Autodesk Fusion 360 part; units mm, degrees
note: some values were not read from the file. Set by a fixed rule: which face or edge a step refers to.
(part 2 of 4)
sketch "Sketch34" plane through (0, 155, 0) normal (0, 1, 0) x (-1, 0, 0)
  line L0 (236, 20) -> (236, 10)
  line L1 (236, 10) -> (241, 10)
  line L2 (241, 10) -> (241, 15)
  line L3 (241, 15) -> (247, 15)
  line L4 (247, 15) -> (247, 10)
  line L5 (247, 10) -> (254, 10)
  line L6 (254, 10) -> (254, 51.2)
  line L7 (254, 51.2) -> (218, 51.2)
  line L8 (218, 51.2) -> (218, 42.3)
  line L9 (218, 42.3) -> (213, 42.3)
  line L10 (213, 42.3) -> (213, 37.3)
  line L11 (213, 37.3) -> (223, 37.3)
  line L12 (223, 37.3) -> (223, 20)
  line L13 (223, 20) -> (236, 20)
  line L14 (223, 20) -> (254, 20)
  line L15 (254, 20) -> (254, 51.2)
  line L16 (254, 51.2) -> (223, 51.2)
  line L17 (223, 51.2) -> (223, 20)
  line L18 (223, 51.2) -> (254, 51.2)
  line L19 (254, 51.2) -> (254, 46.2)
  line L20 (254, 46.2) -> (223, 46.2)
  line L21 (223, 46.2) -> (223, 51.2)
  line L22 (223, 20) -> (254, 20)
  line L23 (254, 20) -> (254, 30.7)
  line L24 (254, 30.7) -> (223, 30.7)
  line L25 (223, 30.7) -> (223, 20)
  line L26 (223, 51.2) -> (228.5, 51.2)
  line L27 (228.5, 51.2) -> (228.5, 20)
  line L28 (228.5, 20) -> (223, 20)
  line L29 (223, 20) -> (223, 51.2)
  line L30 (254, 51.2) -> (248.5, 51.2)
  line L31 (248.5, 51.2) -> (248.5, 20)
  line L32 (248.5, 20) -> (254, 20)
  line L33 (254, 20) -> (254, 51.2)
  dimension "d246" = 5
  dimension "d247" = 31
  dimension "d248" = 10.7
  dimension "d249" = 5.5
  dimension "d250" = 5.5
  constraint horizontal L14
  constraint vertical L15
  constraint horizontal L16
  constraint vertical L17
  constraint coincident L6.end L7.start
  constraint coincident L12.end L13.start
  constraint horizontal L18
  constraint vertical L19
  constraint horizontal L20
  constraint vertical L21
  constraint horizontal L22
  constraint vertical L23
  constraint horizontal L24
  constraint vertical L25
  constraint horizontal L26
  constraint vertical L27
  constraint horizontal L28
  constraint vertical L29
  constraint horizontal L30
  constraint vertical L31
  constraint horizontal L32
  constraint vertical L33
  measures "d246" distance of L16.end L20.end
  measures "d247" distance of L12.end L14.end
  measures "d248" distance of L12.end L24.end
  measures "d249" distance of L16.end L26.end
  measures "d250" distance of L6.end L30.end
extrude "Extrude92" cut sketch "Sketch34" against normal blind 2 contours L20 L24 L27 L31 bodies 1
sketch "Sketch35" plane through (0, 155, 0) normal (0, 1, 0) x (-1, 0, 0)
  line L0 (228.5, 46.2) -> (248.5, 46.2)
  line L1 (248.5, 46.2) -> (248.5, 30.7)
  line L2 (248.5, 30.7) -> (228.5, 30.7)
  line L3 (228.5, 30.7) -> (228.5, 46.2)
  line L4 (236, 20) -> (236, 10)
  line L5 (236, 10) -> (241, 10)
  line L6 (241, 10) -> (241, 15)
  line L7 (241, 15) -> (247, 15)
  line L8 (247, 15) -> (247, 10)
  line L9 (247, 10) -> (254, 10)
  line L10 (254, 10) -> (254, 51.2)
  line L11 (254, 51.2) -> (218, 51.2)
  line L12 (218, 51.2) -> (218, 42.3)
  line L13 (218, 42.3) -> (213, 42.3)
  line L14 (213, 42.3) -> (213, 37.3)
  line L15 (213, 37.3) -> (223, 37.3)
  line L16 (223, 37.3) -> (223, 20)
  line L17 (223, 20) -> (236, 20)
  line L18 (226.5, 48.2) -> (250.5, 48.2)
  line L19 (250.5, 48.2) -> (250.5, 28.7)
  line L20 (250.5, 28.7) -> (226.5, 28.7)
  line L21 (226.5, 28.7) -> (226.5, 48.2)
  dimension "d253" = -2
extrude "Extrude93" cut sketch "Sketch35" against normal blind 1 contours L18 L19 L20 L21 bodies 1
extrude "Extrude94" add 1 faces at (-236, 150, 36.1667) along direction (0, -1, 0) blind 5 on bodies 1 bodies 1
sketch "Sketch36" plane through (0, 153, 0) normal (0, 1, 0) x (-1, 0, 0)
  line L0 (248.5, 30.7) -> (248.5, 46.2)
  line L1 (248.5, 46.2) -> (228.5, 46.2)
  line L2 (228.5, 46.2) -> (228.5, 30.7)
  line L3 (228.5, 30.7) -> (248.5, 30.7)
  line L4 (228.5, 30.7) -> (248.5, 30.7)
  line L5 (248.5, 30.7) -> (248.5, 42.7)
  line L6 (248.5, 42.7) -> (228.5, 42.7)
  line L7 (228.5, 42.7) -> (228.5, 30.7)
  dimension "d258" = 12
  constraint horizontal L4
  constraint vertical L5
  constraint horizontal L6
  constraint vertical L7
  constraint coincident L2.end L3.start
  measures "d258" distance of L2.end L6.end
extrude "Extrude95" cut sketch "Sketch36" against normal blind 8 contours L0 L1 L2 L6 bodies 1
extrude "Extrude96" cut 1 faces at (-235.1667, 148, 46.2) along direction (0, 0, 1) blind 2 on bodies 1 bodies 1
extrude "Extrude97" cut 1 faces at (-235.1667, 148, 48.2) along direction (0, 0, 1) blind 3 on bodies 1 bodies 1
sketch "Sketch37" plane through (0, 153, 0) normal (0, 1, 0) x (-1, 0, 0)
  line L0 (248.5, 42.7) -> (228.5, 42.7)
  line L1 (228.5, 42.7) -> (228.5, 30.7)
  line L2 (228.5, 30.7) -> (248.5, 30.7)
  line L3 (248.5, 30.7) -> (248.5, 42.7)
  line L4 (228.5, 30.7) -> (230, 30.7)
  line L5 (230, 30.7) -> (230, 32.2)
  line L6 (230, 32.2) -> (228.5, 32.2)
  line L7 (228.5, 32.2) -> (228.5, 30.7)
  line L8 (248.5, 30.7) -> (247, 30.7)
  line L9 (247, 30.7) -> (247, 32.2)
  line L10 (247, 32.2) -> (248.5, 32.2)
  line L11 (248.5, 32.2) -> (248.5, 30.7)
  circle A0 centre (230, 32.2) radius 1.5
  circle A1 centre (247, 32.2) radius 1.5
  dimension "d265" = 1.5
  dimension "d266" = 1.5
  dimension "d267" = 1.5
  dimension "d268" = 1.5
  dimension "d269" = 3
  dimension "d270" = 3
  constraint horizontal L4
  constraint vertical L5
  constraint horizontal L6
  constraint vertical L7
  constraint coincident L1.end L2.start
  constraint horizontal L8
  constraint vertical L9
  constraint horizontal L10
  constraint vertical L11
  constraint coincident L2.end L3.start
  constraint coincident L5.end L6.start
  constraint coincident L9.end L10.start
  measures "d265" distance of L1.end L4.end
  measures "d266" distance of L1.end L6.end
  measures "d267" distance of L2.end L8.end
  measures "d268" distance of L2.end L10.end
  measures "d269" diameter of A0
  measures "d270" diameter of A1
extrude "Extrude98" cut sketch "Sketch37" against normal blind 8 contours L9 L10 A1 | L9 L10 A1 | L5 L6 A0 | L5 L6 A0 bodies 1
extrude "Extrude99" cut 1 faces at (-241.8333, 154, 29.3667) along direction (0, -1, 0) blind 4 on bodies 1 bodies 1
extrude "Extrude100" cut 1 faces at (-236.0332, 153, 39.5401) along direction (0, -1, 0) blind 3 on bodies 1 bodies 1
extrude "Extrude101" cut 1 faces at (-248.2053, 153, 30.9947) along direction (0, -1, 0) blind 3 on bodies 1 bodies 1
extrude "Extrude102" cut 1 faces at (-228.7947, 153, 30.9947) along direction (0, -1, 0) blind 3 on bodies 1 bodies 1
sketch "Sketch38" plane through (0, 150, 0) normal (0, 1, 0) x (-1, 0, 0)
  circle A0 centre (247, 32.2) radius 1.5
  circle A1 centre (230, 32.2) radius 1.5
  line L0 (248.5, 42.7) -> (228.5, 42.7)
  line L1 (228.5, 42.7) -> (228.5, 51.2)
  line L2 (228.5, 51.2) -> (226.5, 51.2)
  line L3 (226.5, 51.2) -> (226.5, 28.7)
  line L4 (226.5, 28.7) -> (250.5, 28.7)
  line L5 (250.5, 28.7) -> (250.5, 51.2)
  line L6 (250.5, 51.2) -> (248.5, 51.2)
  line L7 (248.5, 51.2) -> (248.5, 42.7)
  circle A2 centre (230, 32.2) radius 2.5
  circle A3 centre (247, 32.2) radius 2.5
  dimension "d281" = 1
  dimension "d282" = 1
extrude "Extrude103" add sketch "Sketch38" along normal blind 1 contours A2 | A3 bodies 1
extrude "Extrude104" add 1 faces at (-237.6667, 145, 27.6994) along direction (0, -1, 0) blind 10 on bodies 1 bodies 1
extrude "Extrude105" cut 1 faces at (-240.8138, 150, 39.8515) along direction (0, -1, 0) blind 5 on bodies 1 bodies 1
extrude "Extrude106" cut 1 faces at (-240.8138, 145, 39.8515) along direction (0, -1, 0) blind 3 on bodies 1 bodies 1
extrude "Extrude107" cut 1 faces at (-229.0289, 151, 34.1304) along direction (0, -1, 0) blind 5 on bodies 1 bodies 1
extrude "Extrude108" cut 1 faces at (-246.0289, 151, 30.2696) along direction (0, -1, 0) blind 5 on bodies 1 bodies 1
extrude "Extrude109" add 1 faces at (-70.3333, 62, -59.3333) along direction (0, -1, 0) blind 27 on bodies 1 bodies 1
extrude "Extrude110" add 1 faces at (-240.3333, 62, -59.3333) along direction (0, -1, 0) blind 27 on bodies 1 bodies 1
sketch "Sketch39" plane through (0, 0, -61) normal (0, 0, 1) x (1, 0, 0)
  line L0 (-249, 5) -> (-66, 5)
  line L1 (-66, 5) -> (-66, 35)
  line L2 (-66, 35) -> (-79, 35)
  line L3 (-79, 35) -> (-236, 35)
  line L4 (-236, 35) -> (-249, 35)
  line L5 (-249, 35) -> (-249, 5)
  line L6 (-249, 5) -> (-236, 5)
  line L7 (-236, 5) -> (-236, 35)
  line L8 (-236, 35) -> (-249, 35)
  line L9 (-249, 35) -> (-249, 5)
  constraint horizontal L6
  constraint vertical L7
  constraint horizontal L8
  constraint vertical L9
  constraint coincident L3.end L4.start
  constraint coincident L0.start L5.end
extrude "Extrude111" add sketch "Sketch39" along normal blind 5 contours L0 L4 L5 L6 L7 L8 L9 bodies 1
sketch "Sketch40" plane through (0, 0, -61) normal (0, 0, 1) x (1, 0, 0)
  line L0 (-236, 35) -> (-236, 5)
  line L1 (-236, 5) -> (-66, 5)
  line L2 (-66, 5) -> (-66, 35)
  line L3 (-66, 35) -> (-79, 35)
  line L4 (-79, 35) -> (-236, 35)
  line L5 (-66, 5) -> (-79, 5)
  line L6 (-79, 5) -> (-79, 35)
  line L7 (-79, 35) -> (-66, 35)
  line L8 (-66, 35) -> (-66, 5)
  constraint horizontal L5
  constraint vertical L6
  constraint horizontal L7
  constraint vertical L8
  constraint coincident L3.end L4.start
  constraint coincident L1.end L2.start
extrude "Extrude112" add sketch "Sketch40" along normal blind 5 contours L1 L2 L3 L5 L6 L7 L8 bodies 1
extrude "Extrude113" add 1 faces at (-74.6667, 62, 13.3333) along direction (0, -1, 0) blind 57 on bodies 1 bodies 1
sketch "Sketch41" plane through (0, 60.5, 0) normal (0, -1, 0) x (1, 0, 0)
  line L0 (-223, 37.3) -> (-213, 37.3)
  line L1 (-213, 37.3) -> (-213, 45.2)
  line L2 (-213, 45.2) -> (-102, 45.2)
  line L3 (-102, 45.2) -> (-102, 37.3)
  line L4 (-102, 37.3) -> (-92, 37.3)
  line L5 (-92, 37.3) -> (-92, 51.2)
  line L6 (-92, 51.2) -> (-223, 51.2)
  line L7 (-223, 51.2) -> (-223, 37.3)
  line L8 (-92, 51.2) -> (-102, 51.2)
  line L9 (-102, 51.2) -> (-102, 37.3)
  line L10 (-102, 37.3) -> (-92, 37.3)
  line L11 (-92, 37.3) -> (-92, 51.2)
  constraint horizontal L8
  constraint vertical L9
  constraint horizontal L10
  constraint vertical L11
  constraint coincident L3.end L4.start
  constraint coincident L5.end L6.start
extrude "Extrude114" add sketch "Sketch41" along normal blind 2 contours L3 L4 L5 L6 L8 L9 L10 L11 bodies 1
extrude "Extrude115" add 1 faces at (-98.6667, 58.5, 41.9333) along direction (0, -1, 0) blind 53.5 on bodies 1 bodies 1
sketch "Sketch42" plane through (0, 60.5, 0) normal (0, -1, 0) x (1, 0, 0)
  line L0 (-102, 45.2) -> (-102, 51.2)
  line L1 (-102, 51.2) -> (-223, 51.2)
  line L2 (-223, 51.2) -> (-223, 37.3)
  line L3 (-223, 37.3) -> (-213, 37.3)
  line L4 (-213, 37.3) -> (-213, 45.2)
  line L5 (-213, 45.2) -> (-102, 45.2)
  line L6 (-223, 51.2) -> (-213, 51.2)
  line L7 (-213, 51.2) -> (-213, 37.3)
  line L8 (-213, 37.3) -> (-223, 37.3)
  line L9 (-223, 37.3) -> (-223, 51.2)
  line L10 (-213, 51.2) -> (-218, 51.2)
  line L11 (-218, 51.2) -> (-218, 37.3)
  line L12 (-218, 37.3) -> (-213, 37.3)
  line L13 (-213, 37.3) -> (-213, 51.2)
  constraint horizontal L6
  constraint vertical L7
  constraint horizontal L8
  constraint vertical L9
  constraint coincident L3.end L4.start
  constraint coincident L1.end L2.start
  constraint horizontal L10
  constraint vertical L11
  constraint horizontal L12
  constraint vertical L13
  constraint midpoint L3 L11.end
extrude "Extrude116" add sketch "Sketch42" along normal blind 55.5 contours L1 L3 L4 L6 L7 L8 L10 L11 L12 L13 bodies 1
extrude "Extrude117" add 1 faces at (-240.3333, 62, 13.3333) along direction (0, -1, 0) blind 57 on bodies 1 bodies 1
extrude "Extrude118" cut 1 faces at (-228.5, 139.6667, 48.3667) along direction (1, 0, 0) blind 2 on bodies 1 bodies 1
extrude "Extrude119" cut 1 faces at (-248.5, 137.3333, 48.3667) along direction (-1, 0, 0) blind 2 on bodies 1 bodies 1
extrude "Extrude120" cut 1 faces at (-249, 48.3333, 37.9667) along direction (-1, 0, 0) blind 1.5 on bodies 1 bodies 1
sketch "Sketch43" plane through (0, 0, -66) normal (0, 0, -1) x (-1, 0, 0)
  line L0 (56, 160) -> (56, 0)
  line L1 (56, 0) -> (259, 0)
  line L2 (259, 0) -> (259, 160)
  line L3 (259, 160) -> (254, 160)
  line L4 (254, 160) -> (254, 155)
  line L5 (254, 155) -> (236, 155)
  line L6 (236, 155) -> (236, 35)
  line L7 (236, 35) -> (79, 35)
  line L8 (79, 35) -> (79, 155)
  line L9 (79, 155) -> (61, 155)
  line L10 (61, 155) -> (61, 160)
  line L11 (61, 160) -> (56, 160)
extrude "Extrude121" add sketch "Sketch43" along normal blind 5 bodies 1
sketch "Sketch44" plane through (0, 35, 0) normal (0, 1, 0) x (-1, 0, 0)
  line L0 (236, -71) -> (236, -61)
  line L1 (236, -61) -> (79, -61)
  line L2 (79, -61) -> (79, -71)
  line L3 (79, -71) -> (236, -71)
  line L4 (79, -61) -> (236, -61)
  line L5 (236, -61) -> (236, -66)
  line L6 (236, -66) -> (79, -66)
  line L7 (79, -66) -> (79, -61)
  constraint horizontal L4
  constraint vertical L5
  constraint horizontal L6
  constraint vertical L7
  constraint midpoint L0 L5.end
  constraint coincident L1.end L2.start
extrude "Extrude122" cut sketch "Sketch44" against normal blind 10 contours L0 L2 L3 L6 bodies 1
sketch "Sketch45" plane through (0, 0, 0) normal (0, -1, 0) x (1, 0, 0)
  circle A0 through (-148, -53.875, -5) (-154, -50.4109, -5) (-154, -57.3391, -5)
  circle A1 through (-159, -12.125, -5) (-165, -8.6609, -5) (-165, -15.5891, -5)
sketch "Sketch46" plane through (0, 0, 56.2) normal (0, 0, 1) x (1, 0, 0)
  circle A0 centre (-229, 25) radius 5.65
  circle A1 centre (-157.5, 25) radius 5.5
  line L0 (-259, 5) -> (-272.5, 5)
  line L1 (-272.5, 5) -> (-272.5, 0)
  line L2 (-272.5, 0) -> (-42.5, 0)
  line L3 (-42.5, 0) -> (-42.5, 5)
  line L4 (-42.5, 5) -> (-56, 5)
  line L5 (-56, 5) -> (-56, 160)
  line L6 (-56, 160) -> (-259, 160)
  line L7 (-259, 160) -> (-259, 5)
  circle A2 centre (-229, 25) radius 6.15
  circle A3 centre (-157.5, 25) radius 6.15
  dimension "d323" = 12.3
  dimension "d324" = 12.3
  constraint concentric A0 A2
  constraint concentric A1 A3
  measures "d323" diameter of A2
  measures "d324" diameter of A3
extrude "Extrude123" cut sketch "Sketch46" against normal blind 5 contours A2 | A3 bodies 1
extrude "Extrude124" cut 1 faces at (-183.6667, 15, -61) along direction (0, 0, -1) blind 3 on bodies 1 bodies 1
extrude "Extrude125" cut 1 faces at (-102, 23.5, 44.5667) along direction (1, 0, 0) blind 0.5 on bodies 1 bodies 1
extrude "Extrude126" cut 1 faces at (-213, 23.5, 44.5667) along direction (-1, 0, 0) blind 0.5 on bodies 1 bodies 1
extrude "Extrude127" cut 1 faces at (-215, 95.3333, 42.3) along direction (0, 0, -1) blind 0.5 on bodies 1 bodies 1
extrude "Extrude128" cut 1 faces at (-100, 125.1667, 42.3) along direction (0, 0, -1) blind 0.5 on bodies 1 bodies 1
sketch "Sketch47" plane through (0, 0, -71) normal (0, 0, -1) x (-1, 0, 0)
  line L0 (236, 155) -> (236, 25)
  line L1 (236, 25) -> (79, 25)
  line L2 (79, 25) -> (79, 155)
  line L3 (79, 155) -> (61, 155)
  line L4 (61, 155) -> (61, 160)
  line L5 (61, 160) -> (56, 160)
  line L6 (56, 160) -> (56, 0)
  line L7 (56, 0) -> (259, 0)
  line L8 (259, 0) -> (259, 160)
  line L9 (259, 160) -> (254, 160)
  line L10 (254, 160) -> (254, 155)
  line L11 (254, 155) -> (236, 155)
  line L12 (61, 155) -> (79, 155)
  line L13 (79, 155) -> (79, 25)
  line L14 (79, 25) -> (61, 25)
  line L15 (61, 25) -> (61, 155)
  line L16 (236, 25) -> (254, 25)
  line L17 (254, 25) -> (254, 155)
  line L18 (254, 155) -> (236, 155)
  line L19 (236, 155) -> (236, 25)
  constraint horizontal L12
  constraint vertical L13
  constraint horizontal L14
  constraint vertical L15
  constraint coincident L1.end L2.start
  constraint coincident L3.end L4.start
  constraint horizontal L16
  constraint vertical L17
  constraint horizontal L18
  constraint vertical L19
  constraint coincident L10.end L11.start
  constraint coincident L0.end L1.start
extrude "Extrude129" cut sketch "Sketch47" against normal blind 5 contours L0 L11 L16 L17 L18 L19 | L2 L3 L12 L13 L14 L15 bodies 1
extrude "Extrude130" cut 1 faces at (-97, 95.3333, 44.9333) along direction (1, 0, 0) blind 1 on bodies 1 bodies 1
extrude "Extrude131" cut 1 faces at (-218, 95.3333, 44.9333) along direction (-1, 0, 0) blind 1 on bodies 1 bodies 1
extrude "Extrude132" add 1 faces at (-92, 105, 41.9333) along direction (1, 0, 0) blind 3 on bodies 1 bodies 1
extrude "Extrude133" cut 1 faces at (-138.8333, 65.5, 49.2) along direction (0, -1, 0) blind 1 on bodies 1 bodies 1
extrude "Extrude134" add 1 faces at (-138.8333, 60.5, 49.2) along direction (0, -1, 0) blind 1 on bodies 1 bodies 1
extrude "Extrude135" cut 1 faces at (-70, 125.6667, 15) along direction (0, 0, 1) blind 0.5 on bodies 1 bodies 1
extrude "Extrude136" cut 1 faces at (-70, 96.3333, -61) along direction (0, 0, -1) blind 0.5 on bodies 1 bodies 1
extrude "Extrude137" cut 1 faces at (-245, 96.3333, 15) along direction (0, 0, 1) blind 0.5 on bodies 1 bodies 1
extrude "Extrude138" cut 1 faces at (-243, 128.3333, -61) along direction (0, 0, -1) blind 0.5 on bodies 1 bodies 1
sketch "Sketch48" plane through (0, 5, 0) normal (0, 1, 0) x (-1, 0, 0)
  line L0 (101.5, 37.3) -> (89, 37.3)
  line L1 (89, 37.3) -> (89, 51.2)
  line L2 (89, 51.2) -> (66, 51.2)
  line L3 (66, 51.2) -> (66, 20)
  line L4 (66, 20) -> (79, 20)
  line L5 (79, 20) -> (79, 10)
  line L6 (79, 10) -> (66, 10)
  line L7 (66, 10) -> (66, -20)
  line L8 (66, -20) -> (249, -20)
  line L9 (249, -20) -> (249, 10)
  line L10 (249, 10) -> (236, 10)
  line L11 (236, 10) -> (236, 20)
  line L12 (236, 20) -> (250.5, 20)
  line L13 (250.5, 20) -> (250.5, 51.2)
  line L14 (250.5, 51.2) -> (218, 51.2)
  line L15 (218, 51.2) -> (218, 37.3)
  line L16 (218, 37.3) -> (213.5, 37.3)
  line L17 (213.5, 37.3) -> (213.5, 51.2)
  line L18 (213.5, 51.2) -> (185, 51.2)
  line L19 (185, 51.2) -> (185, 3)
  line L20 (185, 3) -> (130, 3)
  line L21 (130, 3) -> (130, 51.2)
  line L22 (130, 51.2) -> (101.5, 51.2)
  line L23 (101.5, 51.2) -> (101.5, 37.3)
  circle A0 centre (163, -12.125) radius 4
extrude "Extrude139" add 1 faces at (-42.5, 3.3333, 38.4667) along direction (1, 0, 0) blind 42.5 on bodies 1 bodies 1
extrude "Extrude140" add 1 faces at (-272.5, 1.6667, 20.7333) along direction (-1, 0, 0) blind 42.5 on bodies 1 bodies 1
sketch "Sketch49" plane through (0, 0, 3) normal (0, 0, -1) x (-1, 0, 0)
  line L0 (259, 0) -> (185, 0)
  line L1 (185, 0) -> (185, -3)
  line L2 (185, -3) -> (270, -3)
  line L3 (270, -3) -> (270, 0)
  line L4 (270, 0) -> (315, 0)
  line L5 (315, 0) -> (315, 5)
  line L6 (315, 5) -> (259, 5)
  line L7 (259, 5) -> (259, 0)
  line L8 (259, 5) -> (315, 5)
  line L9 (315, 5) -> (315, 0)
  line L10 (315, 0) -> (259, 0)
  line L11 (259, 0) -> (259, 5)
  constraint horizontal L8
  constraint vertical L9
  constraint horizontal L10
  constraint vertical L11
  constraint coincident L4.end L5.start
  constraint coincident L6.end L7.start
extrude "Extrude141" add sketch "Sketch49" along normal blind 3 contours L4 L5 L6 L7 L8 L9 L10 L11 bodies 1
sketch "Sketch50" plane through (0, 0, 3) normal (0, 0, -1) x (-1, 0, 0)
  line L0 (45, 0) -> (45, -3)
  line L1 (45, -3) -> (130, -3)
  line L2 (130, -3) -> (130, 0)
  line L3 (130, 0) -> (56, 0)
  line L4 (56, 0) -> (56, 5)
  line L5 (56, 5) -> (0, 5)
  line L6 (0, 5) -> (0, 0)
  line L7 (0, 0) -> (45, 0)
  line L8 (56, 5) -> (0, 5)
  line L9 (0, 5) -> (0, 0)
  line L10 (0, 0) -> (56, 0)
  line L11 (56, 0) -> (56, 5)
  constraint horizontal L8
  constraint vertical L9
  constraint horizontal L10
  constraint vertical L11
  constraint coincident L6.end L7.start
  constraint coincident L4.end L5.start
extrude "Extrude142" add sketch "Sketch50" along normal blind 3 contours L4 L5 L6 L7 L8 L9 L10 L11 bodies 1
sketch "Sketch51" plane through (0, 5, 0) normal (0, 1, 0) x (-1, 0, 0)
  line L0 (56, 0) -> (56, 56.2)
  line L1 (56, 56.2) -> (0, 56.2)
  line L2 (0, 56.2) -> (0, 0)
  line L3 (0, 0) -> (56, 0)
  line L4 (56, 56.2) -> (0, 0)
  line L5 (56, 56.2) -> (0, 56.2)
  line L6 (0, 56.2) -> (0, 0)
  constraint coincident L0.end L1.start
  constraint coincident L2.end L3.start
  constraint coincident L1.end L2.start
extrude "Extrude143" cut sketch "Sketch51" against normal blind 5 contours L1 L2 L4 L5 L6 bodies 1
sketch "Sketch52" plane through (0, 5, 0) normal (0, 1, 0) x (-1, 0, 0)
  line L0 (315, 0) -> (315, 56.2)
  line L1 (315, 56.2) -> (259, 56.2)
  line L2 (259, 56.2) -> (259, 0)
  line L3 (259, 0) -> (315, 0)
  line L4 (315, 0) -> (259, 56.2)
  line L5 (315, 0) -> (315, 56.2)
  line L6 (315, 56.2) -> (259, 56.2)
  constraint coincident L0.start L3.end
  constraint coincident L1.end L2.start
  constraint coincident L0.end L1.start
extrude "Extrude144" cut sketch "Sketch52" against normal blind 5 contours L0 L1 L4 L5 L6 bodies 1
sketch "Sketch53" plane through (0, 0, 0) normal (0, -1, 0) x (1, 0, 0)
sketch "Sketch54" plane through (0, 5, 0) normal (0, 1, 0) x (-1, 0, 0)
  line L0 (56, 56.2) -> (0, 0)
  line L1 (0, 0) -> (56, 0)
  line L2 (56, 0) -> (56, 56.2)
  line L3 (45, 45.1607, -5) -> (45, 51.2, -5)
  line L4 (45, 51.2, -5) -> (45, 51.2, 0)
  line L5 (45, 51.2) -> (45, 45.1607)
  line L6 (45, 45.1607, 0) -> (45, 45.1607, -5)
  point P0 (45, 45.1607)
  dimension "d369" = 5
  constraint vertical L5
  constraint coincident P0 L5.end
  measures "d369" distance of P0 L5.end
extrude "Extrude145" cut sketch "Sketch54" along normal blind 6 contours L3 L4 L5 L6 in plane through (-45, 5, 0) normal (-1, 0, 0) bodies 1
extrude "Extrude146" add 1 faces at (-47, 3.3333, 45.1607) along direction (0, 0, 1) blind 11 on bodies 1 bodies 1
sketch "Sketch55" plane through (0, 5, 0) normal (0, 1, 0) x (-1, 0, 0)
  line L0 (51, 51.1821) -> (51, 56.1607)
  line L1 (51, 56.1607) -> (45, 56.1607)
  line L2 (45, 56.1607) -> (45, 45.1607)
  line L3 (45, 45.1607) -> (0, 0)
  line L4 (0, 0) -> (56, 0)
  line L5 (56, 0) -> (56, 56.2)
  line L6 (56, 56.2) -> (51, 51.1821)
  line L7 (56, 56.2) -> (51, 56.1607)
  line L8 (51, 51.1821) -> (56, 56.2)
  line L9 (51, 56.1607) -> (51, 51.1821)
  constraint coincident L5.end L6.start
  constraint coincident L0.end L1.start
  constraint coincident L0.start L6.end
extrude "Extrude147" add sketch "Sketch55" against normal blind 5 contours L0 L6 L7 L8 L9 bodies 1
sketch "Sketch56" plane through (-158.0615, 0, 157.499) normal (-0.708366, 0, 0.705845) x (0.705845, 0, 0.708366)
  line L0 (-143.0037, 5) -> (-222.3412, 5)
  line L1 (-222.3412, 5) -> (-222.3412, 0)
  line L2 (-222.3412, 0) -> (-158.5879, 0)
  line L3 (-158.5879, 0) -> (-150.0622, 0)
  line L4 (-150.0622, 0) -> (-143.0037, 0)
  line L5 (-143.0037, 0) -> (-143.0037, 5)
  line L6 (-158.5879, 0, 0) -> (-154.3099, 0, 4.2628)
  line L7 (-154.3099, 0, 4.2628) -> (-150.0622, 0, 0)
  line L8 (-158.5879, 0) -> (-150.0622, 0)
  line L9 (-150.0622, 0) -> (-158.5879, 0)
  line L10 (-158.5879, 0) -> (-158.5879, 5)
  line L11 (-158.5879, 5) -> (-150.0622, 5)
  line L12 (-150.0622, 5) -> (-150.0622, 0)
  point P0 (-154.3099, 0)
  constraint coincident L2.end L3.start
  constraint coincident L3.end L4.start
  constraint horizontal L9
  constraint vertical L10
  constraint horizontal L11
  constraint vertical L12
  constraint coincident L0 L10.end
extrude "Extrude148" add sketch "Sketch56" along normal blind 5 contours L3 L6 L7 L8 L9 in plane through (-158.0615, 0, 157.499) normal (0, 1, 0) bodies 1
sketch "Sketch57" plane through (0, 5, 0) normal (0, 1, 0) x (-1, 0, 0)
  line L0 (315, 0) -> (270, 45.1607)
  line L1 (270, 45.1607) -> (270, 51.2)
  line L2 (270, 51.2) -> (263.9822, 51.2)
  line L3 (263.9822, 51.2) -> (259, 56.2)
  line L4 (259, 56.2) -> (259, 0)
  line L5 (259, 0) -> (315, 0)
  line L6 (259, 56.2) -> (270, 56.2)
  line L7 (270, 56.2) -> (270, 51.2)
  line L8 (270, 51.2) -> (259, 51.2)
  line L9 (259, 51.2) -> (259, 56.2)
  line L10 (259, 56.2) -> (263.9822, 51.2)
  constraint horizontal L6
  constraint vertical L7
  constraint horizontal L8
  constraint vertical L9
  constraint coincident L1.end L2.start
  constraint coincident L3.end L4.start
  constraint coincident L2.end L3.start
extrude "Extrude149" add sketch "Sketch57" against normal blind 5 contours L2 L3 L6 L7 L8 L10 bodies 1
extrude "Extrude150" add 1 faces at (-33.6667, 5, 15.0536) along direction (0, 1, 0) blind 155 on bodies 1 bodies 1
extrude "Extrude151" add 1 faces at (-281.3333, 5, 15.0536) along direction (0, 1, 0) blind 155 on bodies 1 bodies 1
extrude "Extrude152" cut 1 faces at (-243, 67, 11.8333) along direction (0, -1, 0) blind 5 on bodies 1 bodies 1
extrude "Extrude153" cut 1 faces at (-245, 75, -59.6667) along direction (0, -1, 0) blind 5 on bodies 1 bodies 1
extrude "Extrude154" cut 1 faces at (-72, 67, 11.8333) along direction (0, -1, 0) blind 5 on bodies 1 bodies 1
extrude "Extrude155" cut 1 faces at (-72, 67, -59.6667) along direction (0, -1, 0) blind 5 on bodies 1 bodies 1
extrude "Extrude156" add 1 faces at (-63.3333, 155, -61.1667) along direction (0, 1, 0) blind 62 on bodies 1 bodies 1
extrude "Extrude157" add 1 faces at (-251.6667, 155, -61.1667) along direction (0, 1, 0) blind 62 on bodies 1 bodies 1
sketch "Sketch58" plane through (0, 155, 0) normal (0, 1, 0) x (-1, 0, 0)
  line L0 (68, 10) -> (68, 15.5)
  line L1 (68, 15.5) -> (74, 15.5)
  line L2 (74, 15.5) -> (74, 10)
  line L3 (74, 10) -> (79, 10)
  line L4 (79, 10) -> (79, 20)
  line L5 (79, 20) -> (66, 20)
  line L6 (66, 20) -> (66, 51.2)
  line L7 (66, 51.2) -> (61, 51.2)
  line L8 (61, 51.2) -> (61, 10)
  line L9 (61, 10) -> (68, 10)
  line L10 (79, 20) -> (61, 20)
  line L11 (61, 20) -> (61, 15.5)
  line L12 (61, 15.5) -> (79, 15.5)
  line L13 (79, 15.5) -> (79, 20)
  constraint horizontal L10
  constraint vertical L11
  constraint horizontal L12
  constraint vertical L13
  constraint coincident L8 L11.end
  constraint coincident L4.end L5.start
extrude "Extrude158" add sketch "Sketch58" along normal blind 62 contours L0 L8 L9 L12 | L1 L4 L5 L8 L10 L11 L12 L13 | L2 L3 L4 L12 bodies 1
sketch "Sketch59" plane through (0, 155, 0) normal (0, 1, 0) x (-1, 0, 0)
  line L0 (241, 10) -> (241, 15.5)
  line L1 (241, 15.5) -> (247, 15.5)
  line L2 (247, 15.5) -> (247, 10)
  line L3 (247, 10) -> (254, 10)
  line L4 (254, 10) -> (254, 51.2)
  line L5 (254, 51.2) -> (250.5, 51.2)
  line L6 (250.5, 51.2) -> (250.5, 28.7)
  line L7 (250.5, 28.7) -> (226.5, 28.7)
  line L8 (226.5, 28.7) -> (226.5, 51.2)
  line L9 (226.5, 51.2) -> (219, 51.2)
  line L10 (219, 51.2) -> (219, 41.8)
  line L11 (219, 41.8) -> (213.5, 41.8)
  line L12 (213.5, 41.8) -> (213.5, 37.3)
  line L13 (213.5, 37.3) -> (223, 37.3)
  line L14 (223, 37.3) -> (223, 20)
  line L15 (223, 20) -> (236, 20)
  line L16 (236, 20) -> (236, 10)
  line L17 (236, 10) -> (241, 10)
  line L18 (236, 20) -> (254, 20)
  line L19 (254, 20) -> (254, 15.5)
  line L20 (254, 15.5) -> (236, 15.5)
  line L21 (236, 15.5) -> (236, 20)
  constraint horizontal L18
  constraint vertical L19
  constraint horizontal L20
  constraint vertical L21
  constraint coincident L4 L19.end
  constraint coincident L15.end L16.start
extrude "Extrude159" add sketch "Sketch59" along normal blind 62 contours L0 L16 L17 L20 | L1 L4 L16 L18 L19 L20 L21 | L2 L3 L4 L20 bodies 1
extrude "Extrude160" add 1 faces at (-33.6667, 160, 15.0536) along direction (0, 1, 0) blind 65 on bodies 1 bodies 1
sketch "Sketch60" plane through (0, 225, 0) normal (0, 1, 0) x (-1, 0, 0)
  line L0 (270, 56.2) -> (56, 56.2)
  line L1 (56, 56.2) -> (51, 56.1607)
  line L2 (51, 56.1607) -> (45, 56.1607)
  line L3 (45, 56.1607) -> (45, 45.1607)
  line L4 (45, 45.1607) -> (0, 0)
  line L5 (0, 0) -> (56, 0)
  line L6 (56, 0) -> (56, -71)
  line L7 (56, -71) -> (61, -71)
  line L8 (61, -71) -> (61, 51.2)
  line L9 (61, 51.2) -> (254, 51.2)
  line L10 (254, 51.2) -> (254, -71)
  line L11 (254, -71) -> (259, -71)
  line L12 (259, -71) -> (259, 0)
  line L13 (259, 0) -> (315, 0)
  line L14 (315, 0) -> (270, 45.1607)
  line L15 (270, 45.1607) -> (270, 56.2)
  line L16 (254, 51.2) -> (245, 51.2)
  line L17 (245, 51.2) -> (245, 56.2)
  line L18 (245, 56.2) -> (254, 56.2)
  line L19 (254, 56.2) -> (254, 51.2)
  line L20 (61, 51.2) -> (70, 51.2)
  line L21 (70, 51.2) -> (70, 56.2)
  line L22 (70, 56.2) -> (61, 56.2)
  line L23 (61, 56.2) -> (61, 51.2)
  line L24 (70, 51.2) -> (245, 51.2)
  line L25 (245, 51.2) -> (245, 56.2)
  line L26 (245, 56.2) -> (70, 56.2)
  line L27 (70, 56.2) -> (70, 51.2)
  dimension "d402" = 9
  dimension "d403" = 9
  constraint horizontal L16
  constraint vertical L17
  constraint horizontal L18
  constraint vertical L19
  constraint coincident L9.end L10.start
  constraint horizontal L20
  constraint vertical L21
  constraint horizontal L22
  constraint vertical L23
  constraint coincident L8.end L9.start
  constraint horizontal L24
  constraint vertical L25
  constraint horizontal L26
  constraint vertical L27
  measures "d402" distance of L9.end L16.end
  measures "d403" distance of L8.end L20.end
extrude "Extrude161" cut sketch "Sketch60" against normal blind 10 contours L0 L9 L17 L21 L24 L25 L26 L27 bodies 1
sketch "Sketch61" plane through (0, 0, 56.2) normal (0, 0, 1) x (1, 0, 0)
  line L0 (-70, 225) -> (-70, 215)
  line L1 (-70, 215) -> (-245, 215)
  line L2 (-245, 215) -> (-245, 225)
  line L3 (-245, 225) -> (-270, 225)
  line L4 (-270, 225) -> (-270, 0)
  line L5 (-270, 0) -> (-56, 0)
  line L6 (-56, 0) -> (-56, 225)
  line L7 (-56, 225) -> (-70, 225)
  circle A0 centre (-229, 25) radius 6.15
  circle A1 centre (-157.5, 25) radius 6.15
  line L8 (-245, 215) -> (-70, 215)
  line L9 (-70, 215) -> (-70, 203)
  line L10 (-70, 203) -> (-245, 203)
  line L11 (-245, 203) -> (-245, 215)
  dimension "d406" = 175
  dimension "d407" = 12
  constraint horizontal L8
  constraint vertical L9
  constraint horizontal L10
  constraint vertical L11
  constraint coincident L1.end L2.start
  measures "d406" distance of L1.end L0.end
  measures "d407" distance of L1.end L10.end
sketch "Sketch62" plane through (0, 0, 0) normal (1, 0, 0) x (0, 0, -1)
  line L0 (-56.2, 207.5, -240.5) -> (-56.2, 203, -240.5)
  line L1 (-56.2, 203, -240.5) -> (-56.2, 203, -235.5)
  line L2 (-56.2, 203, -235.5) -> (-56.2, 207.5, -235.5)
  line L3 (-56.2, 207.5, -235.5) -> (-56.2, 207.5, -240.5)
  line L4 (-56.2, 207.5, -74.5) -> (-56.2, 203, -74.5)
  line L5 (-56.2, 203, -74.5) -> (-56.2, 203, -79.5)
  line L6 (-56.2, 203, -79.5) -> (-56.2, 207.5, -79.5)
  line L7 (-56.2, 207.5, -79.5) -> (-56.2, 207.5, -74.5)
  circle A0 through (-56.2, 209.5, -79.5) (-56.2, 206.5, -77.7679) (-56.2, 206.5, -81.2321)
  circle A1 through (-56.2, 209.5, -235.5) (-56.2, 206.5, -233.7679) (-56.2, 206.5, -237.2321)
  point P0 (-56.2, 207.5)
  point P1 (-56.2, 207.5)
  dimension "d412" = 5
  dimension "d413" = 5
  dimension "d414" = 4
  dimension "d415" = 4
  constraint coincident P0 P1
  constraint coincident P1 P0
  measures "d412" distance of P0 P1
  measures "d413" distance of P1 P0
extrude "Extrude162" cut sketch "Sketch62" along normal blind 14 contours L2 L3 A1 | L2 L3 A1 | L6 L7 A0 | L6 L7 A0 in plane through (0, 0, 56.2) normal (0, 0, -1) bodies 1
extrude "Extrude163" add sketch "Sketch61" along normal blind 20 contours L1 L8 L9 L10 L11 bodies 1
extrude "Extrude164" cut 1 faces at (-236.6034, 208.137, 56.2) along direction (0, 0, 1) blind 11 on bodies 1 bodies 1
extrude "Extrude165" cut 1 faces at (-80.6034, 208.137, 56.2) along direction (0, 0, 1) blind 13 on bodies 1 bodies 1
extrude "Extrude166" cut 1 faces at (-236.6034, 208.137, 67.2) along direction (0, 0, 1) blind 20 on bodies 1 bodies 1
extrude "Extrude167" cut 1 faces at (-80.6034, 208.137, 69.2) along direction (0, 0, 1) blind 20 on bodies 1 bodies 1
sketch "Sketch63" plane through (0, 0, 76.2) normal (0, 0, 1) x (1, 0, 0)
  circle A0 centre (-79.5, 207.5) radius 2
  circle A1 centre (-235.5, 207.5) radius 2
extrude "Extrude168" cut 1 faces at (-128.3333, 215, 62.8667) along direction (0, -1, 0) blind 1.5 on bodies 1 bodies 1
sketch "Sketch64" plane through (0, 0, 76.2) normal (0, 0, 1) x (1, 0, 0)
  line L0 (-245, 203) -> (-240, 203)
  line L1 (-240, 203) -> (-240, 213.5)
  line L2 (-240, 213.5) -> (-245, 213.5)
  line L3 (-245, 213.5) -> (-245, 203)
  line L4 (-70, 203) -> (-75, 203)
  line L5 (-75, 203) -> (-75, 213.5)
  line L6 (-75, 213.5) -> (-70, 213.5)
  line L7 (-70, 213.5) -> (-70, 203)
  line L8 (-240, 213.5) -> (-231.5, 213.5)
  line L9 (-231.5, 213.5) -> (-231.5, 203)
  line L10 (-231.5, 203) -> (-240, 203)
  line L11 (-240, 203) -> (-240, 213.5)
  line L12 (-75, 213.5) -> (-83.5, 213.5)
  line L13 (-83.5, 213.5) -> (-83.5, 203)
  line L14 (-83.5, 203) -> (-75, 203)
  line L15 (-75, 203) -> (-75, 213.5)
  point P0 (-245, 203)
  point P1 (-70, 203)
  dimension "d430" = 5
  dimension "d431" = 5
  dimension "d432" = 8.5
  dimension "d433" = 8.5
  constraint horizontal L0
  constraint vertical L1
  constraint horizontal L2
  constraint vertical L3
  constraint coincident P0 L0.start
  constraint horizontal L4
  constraint vertical L5
  constraint horizontal L6
  constraint vertical L7
  constraint coincident P1 L4.start
  constraint horizontal L8
  constraint vertical L9
  constraint horizontal L10
  constraint vertical L11
  constraint horizontal L12
  constraint vertical L13
  constraint horizontal L14
  constraint vertical L15
  measures "d430" distance of P0 L0.end
  measures "d431" distance of P1 L4.end
  measures "d432" distance of L1.end L8.end
  measures "d433" distance of L5.end L12.end
extrude "Extrude169" cut sketch "Sketch64" against normal blind 5 contours L1 L8 L9 L10 L11 | L5 L12 L13 L14 L15 bodies 1
sketch "Sketch65" plane through (0, 0, 51.2) normal (0, 0, -1) x (-1, 0, 0)
  circle A0 centre (229, 25) radius 6.15
  line L0 (245, 225) -> (245, 213.5)
  line L1 (245, 213.5) -> (70, 213.5)
  line L2 (70, 213.5) -> (70, 225)
  line L3 (70, 225) -> (61, 225)
  line L4 (61, 225) -> (61, 155)
  line L5 (61, 155) -> (66, 155)
  line L6 (66, 155) -> (66, 5)
  line L7 (66, 5) -> (89, 5)
  line L8 (89, 5) -> (89, 155)
  line L9 (89, 155) -> (96, 155)
  line L10 (96, 155) -> (96, 64.5)
  line L11 (96, 64.5) -> (219, 64.5)
  line L12 (219, 64.5) -> (219, 155)
  line L13 (219, 155) -> (226.5, 155)
  line L14 (226.5, 155) -> (226.5, 135)
  line L15 (226.5, 135) -> (223, 135)
  line L16 (223, 135) -> (223, 60.5)
  line L17 (223, 60.5) -> (218, 60.5)
  line L18 (218, 60.5) -> (218, 5)
  line L19 (218, 5) -> (250.5, 5)
  line L20 (250.5, 5) -> (250.5, 155)
  line L21 (250.5, 155) -> (254, 155)
  line L22 (254, 155) -> (254, 225)
  line L23 (254, 225) -> (245, 225)
  circle A1 centre (235.5, 207.5) radius 2
  circle A2 centre (79.5, 207.5) radius 2
  line L24 (70, 213.5) -> (245, 213.5)
  line L25 (245, 213.5) -> (245, 317.5)
  line L26 (245, 317.5) -> (70, 317.5)
  line L27 (70, 317.5) -> (70, 213.5)
  line L28 (70, 317.5) -> (245, 317.5)
  line L29 (245, 317.5) -> (245, 328)
  line L30 (245, 328) -> (70, 328)
  line L31 (70, 328) -> (70, 317.5)
  line L32 (61, 225) -> (70, 225)
  line L33 (70, 225) -> (70, 328)
  line L34 (70, 328) -> (61, 328)
  line L35 (61, 328) -> (61, 225)
  line L36 (254, 225) -> (245, 225)
  line L37 (245, 225) -> (245, 328)
  line L38 (245, 328) -> (254, 328)
  line L39 (254, 328) -> (254, 225)
  dimension "d436" = 104
  dimension "d437" = 10.5
  constraint horizontal L24
  constraint vertical L25
  constraint horizontal L26
  constraint vertical L27
  constraint coincident L1.end L2.start
  constraint horizontal L28
  constraint vertical L29
  constraint horizontal L30
  constraint vertical L31
  constraint horizontal L32
  constraint vertical L33
  constraint horizontal L34
  constraint vertical L35
  constraint coincident L3.end L4.start
  constraint horizontal L36
  constraint vertical L37
  constraint horizontal L38
  constraint vertical L39
  constraint coincident L22.end L23.start
  measures "d436" distance of L1.end L26.end
  measures "d437" distance of L26.end L30.end
extrude "Extrude170" add sketch "Sketch65" against normal blind 25 contours L23 L25 L29 L36 L37 L38 L39 | L26 L28 L29 L30 L31 L33 L37 | L3 L27 L31 L32 L33 L34 L35 bodies 1
sketch "Sketch66" plane through (0, 0, 56.2) normal (0, 0, 1) x (1, 0, 0)
  circle A0 centre (-157.5, 25) radius 6.15
  circle A1 centre (-229, 25) radius 6.15
  line L0 (-70, 225) -> (-70, 213.5)
  line L1 (-70, 213.5) -> (-70, 203)
  line L2 (-70, 203) -> (-245, 203)
  line L3 (-245, 203) -> (-245, 213.5)
  line L4 (-245, 213.5) -> (-245, 225)
  line L5 (-245, 225) -> (-254, 225)
  line L6 (-254, 225) -> (-270, 225)
  line L7 (-270, 225) -> (-270, 0)
  line L8 (-270, 0) -> (-56, 0)
  line L9 (-56, 0) -> (-56, 225)
  line L10 (-56, 225) -> (-61, 225)
  line L11 (-61, 225) -> (-70, 225)
  line L12 (-245, 203) -> (-254, 203)
  line L13 (-254, 203) -> (-254, 225)
  line L14 (-254, 225) -> (-245, 225)
  line L15 (-245, 225) -> (-245, 203)
  line L16 (-61, 225) -> (-70, 225)
  line L17 (-70, 225) -> (-70, 203)
  line L18 (-70, 203) -> (-61, 203)
  line L19 (-61, 203) -> (-61, 225)
  constraint horizontal L12
  constraint vertical L13
  constraint horizontal L14
  constraint vertical L15
  constraint coincident L5.end L6.start
  constraint coincident L2.end L3.start
  constraint horizontal L16
  constraint vertical L17
  constraint horizontal L18
  constraint vertical L19
  constraint coincident L1.end L2.start
  constraint coincident L10.end L11.start
extrude "Extrude171" add sketch "Sketch66" along normal blind 20 contours L0 L1 L11 L16 L17 L18 L19 | L3 L4 L5 L12 L13 L14 L15 bodies 1
sketch "Sketch67" plane through (0, 0, 76.2) normal (0, 0, 1) x (1, 0, 0)
  line L0 (-240, 203) -> (-240, 213.5)
  line L1 (-240, 213.5) -> (-245, 213.5)
  line L2 (-245, 213.5) -> (-245, 317.5)
  line L3 (-245, 317.5) -> (-70, 317.5)
  line L4 (-70, 317.5) -> (-70, 213.5)
  line L5 (-70, 213.5) -> (-75, 213.5)
  line L6 (-75, 213.5) -> (-75, 203)
  line L7 (-75, 203) -> (-61, 203)
  line L8 (-61, 203) -> (-61, 328)
  line L9 (-61, 328) -> (-254, 328)
  line L10 (-254, 328) -> (-254, 203)
  line L11 (-254, 203) -> (-240, 203)
  line L12 (-245, 317.5) -> (-70, 317.5)
  line L13 (-70, 317.5) -> (-70, 328)
  line L14 (-70, 328) -> (-245, 328)
  line L15 (-245, 328) -> (-245, 317.5)
  line L16 (-245, 328) -> (-235.5, 328)
  line L17 (-235.5, 328) -> (-235.5, 323.5)
  line L18 (-235.5, 323.5) -> (-245, 323.5)
  line L19 (-245, 323.5) -> (-245, 328)
  line L20 (-70, 328) -> (-79.5, 328)
  line L21 (-79.5, 328) -> (-79.5, 323.5)
  line L22 (-79.5, 323.5) -> (-70, 323.5)
  line L23 (-70, 323.5) -> (-70, 328)
  circle A0 centre (-235.5, 323.5) radius 2
  circle A1 centre (-79.5, 323.5) radius 2
  dimension "d442" = 9.5
  dimension "d443" = 4.5
  dimension "d444" = 9.5
  dimension "d445" = 4.5
  dimension "d446" = 4
  dimension "d447" = 4
  constraint horizontal L12
  constraint vertical L13
  constraint horizontal L14
  constraint vertical L15
  constraint coincident L9 L13.end
  constraint coincident L2.end L3.start
  constraint horizontal L16
  constraint vertical L17
  constraint horizontal L18
  constraint vertical L19
  constraint horizontal L20
  constraint vertical L21
  constraint horizontal L22
  constraint vertical L23
  constraint coincident L17.end L18.start
  constraint coincident L21.end L22.start
  measures "d442" distance of L14.end L16.end
  measures "d443" distance of L14.end L18.end
  measures "d444" distance of L13.end L20.end
  measures "d445" distance of L13.end L22.end
  measures "d446" diameter of A0
  measures "d447" diameter of A1
extrude "Extrude172" cut sketch "Sketch67" against normal blind 25 contours L17 L18 A0 | L17 L18 A0 | L21 L22 A1 | L21 L22 A1 bodies 1
extrude "Extrude173" add 1 faces at (-33.6667, 225, 15.0536) along direction (0, 1, 0) blind 103 on bodies 1 bodies 1
extrude "Extrude174" add 1 faces at (-281.3333, 225, 15.0536) along direction (0, 1, 0) blind 103 on bodies 1 bodies 1
sketch "Sketch68" plane through (0, 328, 0) normal (0, 1, 0) x (-1, 0, 0)
  line L0 (61, 51.2) -> (254, 51.2)
  line L1 (254, 51.2) -> (254, -71)
  line L2 (254, -71) -> (259, -71)
  line L3 (259, -71) -> (259, 0)
  line L4 (259, 0) -> (315, 0)
  line L5 (315, 0) -> (270, 45.1607)
  line L6 (270, 45.1607) -> (270, 56.2)
  line L7 (270, 56.2) -> (254, 56.2)
  line L8 (254, 56.2) -> (254, 76.2)
  line L9 (254, 76.2) -> (61, 76.2)
  line L10 (61, 76.2) -> (61, 56.2)
  line L11 (61, 56.2) -> (56, 56.2)
  line L12 (56, 56.2) -> (51, 56.1607)
  line L13 (51, 56.1607) -> (45, 56.1607)
  line L14 (45, 56.1607) -> (45, 45.1607)
  line L15 (45, 45.1607) -> (0, 0)
  line L16 (0, 0) -> (56, 0)
  line L17 (56, 0) -> (56, -71)
  line L18 (56, -71) -> (61, -71)
  line L19 (61, -71) -> (61, 51.2)
  line L20 (56, 0) -> (36, 0)
  line L21 (36, 0) -> (36, 45.1607)
  line L22 (36, 45.1607) -> (56, 45.1607)
  line L23 (56, 45.1607) -> (56, 0)
  line L24 (259, 0) -> (279, 0)
  line L25 (279, 0) -> (279, 45.1607)
  line L26 (279, 45.1607) -> (259, 45.1607)
  line L27 (259, 45.1607) -> (259, 0)
  dimension "d454" = 20
  dimension "d455" = 20
  constraint horizontal L20
  constraint vertical L21
  constraint horizontal L22
  constraint vertical L23
  constraint coincident L16.end L17.start
  constraint horizontal L24
  constraint vertical L25
  constraint horizontal L26
  constraint vertical L27
  constraint coincident L3.end L4.start
  measures "d454" distance of L16.end L20.end
  measures "d455" distance of L3.end L24.end
extrude "Extrude175" cut sketch "Sketch68" against normal blind 380 contours L15 L16 L21 | L4 L5 L25 bodies 1
sketch "Sketch69" plane through (0, 328, 0) normal (0, 1, 0) x (-1, 0, 0)
  line L0 (36, 36.1286) -> (36, 0)
  line L1 (36, 0) -> (56, 0)
  line L2 (56, 0) -> (56, -71)
  line L3 (56, -71) -> (61, -71)
  line L4 (61, -71) -> (61, 51.2)
  line L5 (61, 51.2) -> (254, 51.2)
  line L6 (254, 51.2) -> (254, -71)
  line L7 (254, -71) -> (259, -71)
  line L8 (259, -71) -> (259, 0)
  line L9 (259, 0) -> (279, 0)
  line L10 (279, 0) -> (279, 36.1286)
  line L11 (279, 36.1286) -> (270, 45.1607)
  line L12 (270, 45.1607) -> (270, 56.2)
  line L13 (270, 56.2) -> (254, 56.2)
  line L14 (254, 56.2) -> (254, 76.2)
  line L15 (254, 76.2) -> (61, 76.2)
  line L16 (61, 76.2) -> (61, 56.2)
  line L17 (61, 56.2) -> (56, 56.2)
  line L18 (56, 56.2) -> (51, 56.1607)
  line L19 (51, 56.1607) -> (45, 56.1607)
  line L20 (45, 56.1607) -> (45, 45.1607)
  line L21 (45, 45.1607) -> (36, 36.1286)
  line L22 (270, 56.2) -> (254, 76.2)
  line L23 (254, 56.2) -> (254, 76.2)
  line L24 (270, 56.2) -> (254, 56.2)
  line L25 (61, 56.2) -> (45, 56.1607)
  line L26 (45, 56.1607) -> (61, 76.2)
  line L27 (61, 76.2) -> (61, 56.2)
  constraint coincident L12.end L13.start
  constraint coincident L14.end L15.start
  constraint coincident L13.end L14.start
  constraint coincident L16.end L17.start
  constraint coincident L19.end L20.start
  constraint coincident L15.end L16.start
extrude "Extrude176" add sketch "Sketch69" against normal blind 328 separate body contours L16 L17 L18 L25 L26 L27 | L13 L14 L22 L23 L24 makes body 2 at (-50.3333, 218.6667, 62.8405) makes body 3 at (-264.6667, 218.6667, 62.8667)
sketch "Sketch70" plane through (-254, 0, 0) normal (1, 0, 0) x (0, 0, -1)
  line L0 (-56.2, 328) -> (-76.2, 328)
  line L1 (-76.2, 328) -> (-76.2, 0)
  line L2 (-76.2, 0) -> (-56.2, 0)
  line L3 (-56.2, 0) -> (-56.2, 328)
  line L4 (-56.2, 0) -> (-76.2, 0)
  line L5 (-76.2, 0) -> (-76.2, 5)
  line L6 (-76.2, 5) -> (-56.2, 5)
  line L7 (-56.2, 5) -> (-56.2, 0)
  dimension "d460" = 5
  constraint horizontal L4
  constraint vertical L5
  constraint horizontal L6
  constraint vertical L7
  constraint coincident L2.end L3.start
  measures "d460" distance of L2.end L6.end
extrude "Extrude177" add sketch "Sketch70" along normal blind 193 contours L1 L2 L3 L4 L5 L6 L7 bodies 1 2 3
sketch "Sketch71" plane through (0, 0, 76.2) normal (0, 0, 1) x (1, 0, 0)
  circle A0 centre (-235.5, 323.5) radius 2
  circle A1 centre (-79.5, 323.5) radius 2
  line L0 (-240, 203) -> (-240, 213.5)
  line L1 (-240, 213.5) -> (-245, 213.5)
  line L2 (-245, 213.5) -> (-245, 317.5)
  line L3 (-245, 317.5) -> (-70, 317.5)
  line L4 (-70, 317.5) -> (-70, 213.5)
  line L5 (-70, 213.5) -> (-75, 213.5)
  line L6 (-75, 213.5) -> (-75, 203)
  line L7 (-75, 203) -> (-61, 203)
  line L8 (-61, 203) -> (-61, 328)
  line L9 (-61, 328) -> (-254, 328)
  line L10 (-254, 328) -> (-254, 203)
  line L11 (-254, 203) -> (-240, 203)
  circle A2 centre (-235.5, 323.5) radius 2
  circle A3 centre (-79.5, 323.5) radius 2
  line L12 (-70, 317.5) -> (-75, 317.5)
  line L13 (-75, 317.5) -> (-75, 328)
  line L14 (-75, 328) -> (-70, 328)
  line L15 (-70, 328) -> (-70, 317.5)
  line L16 (-75, 328) -> (-83.5, 328)
  line L17 (-83.5, 328) -> (-83.5, 317.5)
  line L18 (-83.5, 317.5) -> (-75, 317.5)
  line L19 (-75, 317.5) -> (-75, 328)
  line L20 (-245, 317.5) -> (-240, 317.5)
  line L21 (-240, 317.5) -> (-240, 328)
  line L22 (-240, 328) -> (-245, 328)
  line L23 (-245, 328) -> (-245, 317.5)
  line L24 (-240, 328) -> (-231.5, 328)
  line L25 (-231.5, 328) -> (-231.5, 317.5)
  line L26 (-231.5, 317.5) -> (-240, 317.5)
  line L27 (-240, 317.5) -> (-240, 328)
  dimension "d463" = 5
  dimension "d464" = 8.5
  dimension "d465" = 5
  dimension "d466" = 8.5
  constraint concentric A0 A2
  constraint concentric A1 A3
  constraint horizontal L12
  constraint vertical L13
  constraint horizontal L14
  constraint vertical L15
  constraint coincident L3.end L4.start
  constraint horizontal L16
  constraint vertical L17
  constraint horizontal L18
  constraint vertical L19
  constraint horizontal L20
  constraint vertical L21
  constraint horizontal L22
  constraint vertical L23
  constraint coincident L2.end L3.start
  constraint horizontal L24
  constraint vertical L25
  constraint horizontal L26
  constraint vertical L27
  measures "d463" distance of L3.end L12.end
  measures "d464" distance of L13.end L16.end
  measures "d465" distance of L2.end L20.end
  measures "d466" distance of L21.end L24.end
extrude "Extrude178" cut sketch "Sketch71" against normal blind 5 contours L3 L9 L21 L24 L25 L26 L27 | L3 L9 L13 L16 L17 L18 L19 bodies 1
extrude "Extrude179" cut 1 faces at (-240, 321, 74.5333) along direction (-1, 0, 0) blind 0.5 on bodies 1 bodies 1
extrude "Extrude180" cut 1 faces at (-240, 206.5, 74.5333) along direction (-1, 0, 0) blind 0.5 on bodies 1 bodies 1
extrude "Extrude181" cut 1 faces at (-75, 321, 74.5333) along direction (1, 0, 0) blind 0.5 on bodies 1 bodies 1
extrude "Extrude182" cut 1 faces at (-75, 206.5, 74.5333) along direction (1, 0, 0) blind 0.5 on bodies 1 bodies 1
extrude "Extrude183" cut 1 faces at (-79.1168, 318.8352, 71.2) along direction (0, 0, -1) blind 2.5 on bodies 1 bodies 1
extrude "Extrude184" cut 1 faces at (-235.8832, 318.8352, 71.2) along direction (0, 0, -1) blind 2.5 on bodies 1 bodies 1
extrude "Extrude185" cut 1 faces at (-235.9327, 212.1592, 71.2) along direction (0, 0, -1) blind 2.5 on bodies 1 bodies 1
extrude "Extrude186" cut 1 faces at (-79.0673, 212.1592, 71.2) along direction (0, 0, -1) blind 2.5 on bodies 1 bodies 1
sketch "Sketch72" plane through (-245, 0, 0) normal (1, 0, 0) x (0, 0, -1)
  line L0 (-76.2, 213.5) -> (-51.2, 213.5)
  line L1 (-51.2, 213.5) -> (-51.2, 317.5)
  line L2 (-51.2, 317.5) -> (-76.2, 317.5)
  line L3 (-76.2, 317.5) -> (-76.2, 213.5)
  line L4 (-76.2, 213.5) -> (-69.7, 213.5)
  line L5 (-69.7, 213.5) -> (-69.7, 317.5)
  line L6 (-69.7, 317.5) -> (-76.2, 317.5)
  line L7 (-76.2, 317.5) -> (-76.2, 213.5)
  line L8 (-69.7, 317.5) -> (-62.7, 317.5)
  line L9 (-62.7, 317.5) -> (-62.7, 272.5)
  line L10 (-62.7, 272.5) -> (-69.7, 272.5)
  line L11 (-69.7, 272.5) -> (-69.7, 317.5)
  line L12 (-69.7, 272.5) -> (-59.7, 272.5)
  line L13 (-59.7, 272.5) -> (-59.7, 213.5)
  line L14 (-59.7, 213.5) -> (-69.7, 213.5)
  line L15 (-69.7, 213.5) -> (-69.7, 272.5)
  dimension "d485" = 6.5
  dimension "d486" = 7
  dimension "d487" = 45
  dimension "d488" = 10
  constraint horizontal L4
  constraint vertical L5
  constraint horizontal L6
  constraint vertical L7
  constraint coincident L0.start L3.end
  constraint horizontal L8
  constraint vertical L9
  constraint horizontal L10
  constraint vertical L11
  constraint horizontal L12
  constraint vertical L13
  constraint horizontal L14
  constraint vertical L15
  constraint coincident L0 L13.end
  measures "d485" distance of L0.start L4.end
  measures "d486" distance of L5.end L8.end
  measures "d487" distance of L5.end L10.end
  measures "d488" distance of L10.end L12.end
extrude "Extrude187" cut sketch "Sketch72" against normal blind 30 contours L0 L5 L10 L12 L13 L14 L15 bodies 1
extrude "Extrude188" cut 1 faces at (-257.1333, 272.5, 63.0333) along direction (0, 1, 0) blind 5 on bodies 1 bodies 1